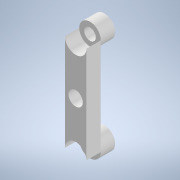
# Autodesk Inventor part: constraining plate
Saved by Autodesk Inventor 2022 (Build 260153000, 153)
## iProperties
Created: 2022-01-15
Part Number: constraining plate
Material: Generic
Document SubType Name: Modeling
Designer: simon
Density: 1 g/cm^3
Appearance: Default
Author: simon
Autodesk Inventor part; units mm, degrees
ref_plane "YZ Plane" through (0, 0, 0) normal (1, 0, 0) x (0, 1, 0)
ref_plane "XZ Plane" through (0, 0, 0) normal (0, 1, 0) x (-1, 0, 0)
ref_plane "XY Plane" through (0, 0, 0) normal (0, 0, 1) x (1, 0, 0)
sketch "Sketch1" plane through (0, 0, 0) normal (0, 0, 1) x (1, 0, 0)
  circle A0 centre (157.7925, 25.2801) radius 7.5 projected
  circle A1 centre (157.7925, 25.2801) radius 4.05 projected
  circle A2 centre (157.7925, -42.1199) radius 7.5 projected
  circle A3 centre (157.7925, -42.1199) radius 4.05 projected
  line L0 (7.5, 7.5) -> (-7.5, 7.5)
  line L1 (-7.5, 7.5) -> (-7.5, -74.9)
  line L2 (-7.5, -74.9) -> (7.5, -74.9)
  line L3 (7.5, -74.9) -> (7.5, 7.5)
  line L4 (7.5, 7.5) -> (-7.5, 7.5)
  line L5 (-7.5, 7.5) -> (-7.5, -74.9)
  line L6 (-7.5, -74.9) -> (7.5, -74.9)
  line L7 (7.5, -74.9) -> (7.5, 7.5)
  circle A4 centre (157.7925, 25.2801) radius 4.05 projected
  circle A5 centre (157.7925, 25.2801) radius 7.5 projected
  circle A6 centre (157.7925, 25.2801) radius 4.05 projected
  circle A7 centre (157.7925, -42.1199) radius 4.05 projected
  circle A8 centre (157.7925, -42.1199) radius 7.5 projected
  circle A9 centre (157.7925, -42.1199) radius 4.05 projected
  line L8 (7.5, 7.5) -> (-7.5, 7.5)
  line L9 (-7.5, 7.5) -> (-7.5, -74.9)
  line L10 (-7.5, -74.9) -> (7.5, -74.9)
  line L11 (7.5, -74.9) -> (7.5, 7.5)
  point P0 (0, 0)
  constraints: 24 end point, 6 parallel, 3 horizontal, 3 perpendicular
extrude "Extrusion1" add sketch "Sketch1" against normal blind 10 contours A0 | A2
sketch "Sketch2" plane through (157.7925, 25.2801, 0) normal (0, 0, 1) x (1, 0, 0)
  line L0 (7.5, 7.5) -> (-7.5, 7.5)
  line L1 (-7.5, 7.5) -> (-7.5, -74.9)
  line L2 (-7.5, -74.9) -> (7.5, -74.9)
  line L3 (7.5, -74.9) -> (7.5, 7.5)
  circle A0 centre (0, 0) radius 7.5 projected
  circle A1 centre (0, 0) radius 4.05 projected
  circle A2 centre (0, -67.4) radius 7.5 projected
  circle A3 centre (0, -67.4) radius 4.05 projected
  circle A4 centre (0, -33.7) radius 7.5
  circle A5 centre (0, -33.7) radius 5
  point P0 (-157.7925, -25.2801)
  point P1 (7.5, 0)
  point P2 (-7.5, 0)
  point P3 (-7.5, -67.4)
  point P4 (7.5, -67.4)
  dimension "d2" = 10
  constraints: 8 end point, 2 centre point, 2 parallel, 1 coincident, 1 horizontal, 1 perpendicular
  measures "d2" diameter of A5
extrude "Extrusion2" add sketch "Sketch2" along normal blind 10 contours L3 A0 L0 | A0 L1 L0 | A0 | L3 A4 L1 A0 | A4 | L3 A2 L1 A4 | A2 | L3 L2 A2 | A2 L2 L1 | A1 | A3
fillet "Fillet1" radius 2 4 edges at (150.2925, -49.6199, 5) (165.2925, -49.6199, 5) (165.2925, 32.7801, 5) (150.2925, 32.7801, 5)
body "Solid1"
